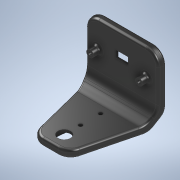
# Autodesk Inventor part: Suporte_Laserv2
Saved by Autodesk Inventor 2020 (Build 240168000, 168)
## iProperties
Created: 2022-06-09
Part Number: Suporte_Laserv2
Material: Genérico
Document SubType Name: Modeling
Designer: JCarlos
Density: 1 g/cm^3
Appearance: Brilhosa - Preta
Author: JCarlos
Autodesk Inventor part; units mm, degrees
ref_plane "YZ Plane" through (0, 0, 0) normal (1, 0, 0) x (0, 1, 0)
sketch "Esboço2" plane through (0, 0, 0) normal (1, 0, 0) x (0, 1, 0)
  line L0 (1.2426, 3) -> (-2.2929, 6.5355)
  line L1 (-2.2929, 6.5355) -> (-2.2929, 31.5355)
  line L2 (1.2426, 3) -> (21.2426, 3)
  line L3 (-5.2929, 31.5355) -> (-5.2929, 5.2929)
  line L4 (-5.2929, 5.2929) -> (0, 0)
  line L5 (0, 0) -> (21.2426, 0)
  line L6 (-5.2929, 31.5355) -> (-2.2929, 31.5355)
  line L7 (21.2426, 3) -> (21.2426, 0)
  dimension "d0" = 135
  dimension "d3" = 5
  dimension "d7" = 25
  dimension "d89" = 135
  dimension "d90" = 20
  dimension "d91" = 3
  dimension "d92" = 3
  constraints: 16 end point, 2 vertical, 1 coincident, 1 horizontal, 1 parallel, 1 other
  measures "d0" angle of L1 L0
  measures "d3" distance of L0.start L0.end
  measures "d7" distance of L0.end L1.end
  measures "d89" angle of L0 L2
  measures "d90" distance of L0.start L2.end
  measures "d91" distance of L3.start L1.end
  measures "d92" distance of L2.end L5.end
extrude "Extrusão1" add sketch "Esboço2" along normal blind 30
sketch "Esboço17" plane through (0, 0, 0) normal (0, 0, -1) x (-1, 0, 0)
  line L0 (-17.5, 14.2426) -> (-12.5, 14.2426)
  line L1 (-12.5, 14.2426) -> (-12.5, 11.2426)
  line L2 (-12.5, 11.2426) -> (-17.5, 11.2426)
  line L3 (-17.5, 11.2426) -> (-17.5, 14.2426)
  line L4 (0, 21.2426) -> (-30, 21.2426) projected
  line L5 (-15, 21.2426) -> (-15, 16.844)
  line L6 (-30, 21.2426) -> (-30, 1.2426) projected
  point P0 (0, 0)
  point P1 (-15, 14.2426)
  dimension "d107" = 5
  dimension "d108" = 3
  dimension "d113" = 7
  constraints: 10 end point, 2 midpoint, 2 parallel, 1 horizontal, 1 perpendicular, 1 vertical, 1 vertical alignment
  measures "d107" distance of L0.start L0.end
  measures "d108" distance of L2.end L0.start
  measures "d113" distance from line of L4.end L0
extrude "Extrusão12" cut sketch "Esboço17" against normal through all
sketch "Esboço8" plane through (0, 1.2426, 3) normal (0, 0, 1) x (1, 0, 0)
  circle A0 centre (5.25, 9.5) radius 1.4
  circle A1 centre (24.75, 9.5) radius 1.4
  line L0 (0, 20) -> (30, 20) projected
  line L1 (15, 20) -> (15, 14.8338)
  line L2 (12.5, 13) -> (12.5, 10) projected
  line L3 (12.5, 11.5) -> (13.8508, 11.5)
  point P0 (0, -1.2426)
  dimension "d36" = 2.8
  dimension "d93" = 19.5
  dimension "d94" = 9.75
  dimension "d112" = 2
  constraints: 4 end point, 2 centre point, 2 midpoint, 1 equal radius, 1 horizontal, 1 horizontal alignment, 1 vertical
  measures "d36" diameter of A0
  measures "d93" distance of A1.centre A0.centre
  measures "d94" horizontal distance of L1.end A0.centre
  measures "d112" vertical distance of A0.centre L3.start
extrude "Extrusão6" add sketch "Esboço8" along normal blind 3
sketch "Esboço10" plane through (5.25, 10.7426, 6) normal (0, 0, 1) x (1, 0, 0)
  circle A0 centre (0, 0) radius 1.4 projected
  point P0 (-5.25, -10.7426)
  constraints: 1 coincident
hole "Furo2" at (5.25, 10.7426, 6) direction (0, 0, -1) diameter 1.5 depth 4
sketch "Esboço12" plane through (0, -5.2929, 5.2929) normal (0, -1, 0) x (1, 0, 0)
  arc A0 (12.7593, 4.0381) -> (17.2407, 4.0381) centre (15, 4.2426) ccw
  line L0 (0, 0) -> (30, 0) projected
  arc A1 (18.7345, 20.4017) -> (11.2655, 20.4017) centre (15, 20.7426) ccw
  line L1 (17.2407, 4.0381) -> (18.7345, 20.4017)
  line L2 (12.7593, 4.0381) -> (11.2655, 20.4017)
  line L3 (0, 26.2426) -> (30, 26.2426) projected
  point P0 (0, -5.2929)
  point P1 (15, 0)
  dimension "d61" = 16.5
  dimension "d62" = 4.5
  dimension "d63" = 7.5
  dimension "d64" = 22
  dimension "d65" = 22.5
  constraints: 4 end point, 4 point on circle, 4 tangent, 2 centre point, 2 vertical alignment, 1 midpoint
  measures "d61" distance of A1.centre A0.centre
  measures "d62" diameter of A0
  measures "d63" diameter of A1
  measures "d64" distance from line of L3 A0.centre
extrude "Extrusão8" cut sketch "Esboço12" against normal blind 2
sketch "Esboço13" plane through (0, -3.2929, 5.2929) normal (0, -1, 0) x (1, 0, 0)
  arc A0 (12.7593, 4.0381) -> (17.2407, 4.0381) centre (15, 4.2426) ccw projected
  circle A1 centre (15, 14.2426) radius 0.75
  circle A2 centre (15, 20.7426) radius 2.5
  arc A3 (18.7345, 20.4017) -> (11.2655, 20.4017) centre (15, 20.7426) ccw projected
  circle A4 centre (15, 6.2426) radius 0.75
  point P0 (0, -5.2929)
  dimension "d82" = 1.5
  dimension "d84" = 5
  dimension "d85" = 1.5
  dimension "d86" = 14.5
  dimension "d87" = 8
  constraints: 3 centre point, 2 vertical alignment, 1 concentric
  measures "d82" diameter of A1
  measures "d84" diameter of A2
  measures "d85" diameter of A4
  measures "d86" distance of A2.centre A4.centre
  measures "d87" distance of A1.centre A4.centre
extrude "Extrusão9" cut sketch "Esboço13" against normal through all
ref_plane "Plano de trabalho1" through (12.5, 0, 0) normal (-1, 0, 0) x (0, 0, 1)
fillet "Arredondamento3" radius 1 2 edges at (3.85, 10.7426, 3) (23.35, 10.7426, 3)
fillet "Arredondamento4" radius 5 4 edges at (15, 0, 0) (15, -5.2929, 5.2929) (15, -2.2929, 6.5355) (15, 1.2426, 3)
sketch "Esboço15" plane through (24.75, 10.7426, 6) normal (0, 0, 1) x (1, 0, 0)
  circle A0 centre (0, 0) radius 1.4 projected
  point P0 (-24.75, -10.7426)
  constraints: 1 coincident
hole "Furo4" at (24.75, 10.7426, 6) direction (0, 0, -1) diameter 1.5 depth 4
sketch "Esboço16" plane through (0, -5.2929, 5.2929) normal (0, -1, 0) x (1, 0, 0)
  line L0 (30, 26.2426) -> (30, 0) projected
  line L1 (30, -5.2929) -> (22, 26.2426)
  line L2 (0, 26.2426) -> (30, 26.2426) projected
  line L3 (30, 1.2426) -> (30, 26.2426) projected
  line L4 (22, 26.2426) -> (30, 26.2426)
  line L5 (30, 26.2426) -> (30, -5.2929)
  point P0 (0, -5.2929)
  point P1 (30, -5.2929)
  point P2 (30, 0)
  dimension "d103" = 8
  constraints: 6 end point, 1 coincident, 1 horizontal, 1 perpendicular, 1 point on line
  measures "d103" distance of L0.start L1.end
extrude "Extrusão11" cut sketch "Esboço16" against normal through all
ref_plane "Plano de trabalho2" through (15, 0, 0) normal (1, 0, 0) x (0, 0, -1)
mirror "Espelhamento2" about plane through (15, 0, 0) normal (1, 0, 0) of "Extrusão11"
fillet "Arredondamento5" radius 5 4 edges at (29.6195, 21.2426, 1.5) (0.3805, 21.2426, 1.5) (22, -3.7929, 31.5355) (8, -3.7929, 31.5355)
fillet "Arredondamento5" radius 1 24 edges at (28.3021, -1.9123, 6.6932) (28.7905, -0.5251, 4.7678) (29.1424, 1.4003, 3.3806) (29.239, 12.2782, 3) (24.9083, -2.2929, 20.0711) (1.6979, -1.9123, 6.6932) (1.2095, -0.5251, 4.7678) (0.8576, 1.4003, 3.3806) (0.761, 12.2782, 3) (5.0917, -2.2929, 20.0711) (15, -2.2929, 31.5355) (15, 21.2426, 3) (29.9034, 0.1577, 0.3806) (29.3286, -2.6464, 2.6464) (28.6173, -4.9123, 5.4505) (25.0659, -5.2929, 19.4497) (30, 11.6569, 0) (15, 21.2426, 0) (0.0966, 0.1577, 0.3806) (0.6714, -2.6464, 2.6464) (1.3827, -4.9123, 5.4505) (4.9341, -5.2929, 19.4497) (0, 11.6569, 0) (15, -5.2929, 31.5355)
chamfer "Chanfro2" distance 2 angle 45 4 edges at (15, 14.2426, 0) (12.5, 12.7426, 0) (15, 11.2426, 0) (17.5, 12.7426, 0)
equation "\"d92\" = d91"
equation "\"d94\" = 0.5 * d93"
equation "\"d106\" = -0.5 * d8"
equation "\"d8\" = 30"
